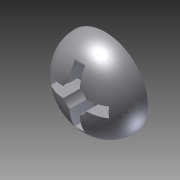
# Autodesk Inventor part: Bolt1
Saved by Autodesk Inventor 2012 SP2 (Build 160219200, 219)
## iProperties
Created: 2014-02-08
Part Number: Bolt1
Material: Default
Document SubType Name: Modeling
Designer: 1
Density: 1 g/cm^3
Author: 1
Autodesk Inventor part; units mm, degrees
ref_plane "YZ Plane" through (0, 0, 0) normal (1, 0, 0) x (0, 1, 0)
ref_plane "XZ Plane" through (0, 0, 0) normal (0, 1, 0) x (-1, 0, 0)
ref_plane "XY Plane" through (0, 0, 0) normal (0, 0, 1) x (1, 0, 0)
sketch "Sketch1" plane through (0, 0, 0) normal (0, 0, 1) x (1, 0, 0)
  circle A0 centre (-3.4351, -7.3738) radius 1.5 projected
  circle A1 centre (-3.4351, -7.3738) radius 4.4749
  point P0 (0, 0)
  constraints: 1 centre point, 1 coincident
extrude "Extrusion1" add sketch "Sketch1" along normal blind 3.175 contours A0 | A1
fillet "Fillet1" radius 3.175 1 edges at (-7.91, -7.3738, 3.175)
sketch "Sketch2" plane through (-3.4351, -7.3738, 3.175) normal (0, 0, 1) x (1, 0, 0)
  circle A0 centre (0, 0) radius 1.2999 construction
  line L0 (-6.0004, 0) -> (5.9052, 0) construction
  line L1 (0.0173, 5.7893) -> (0.0173, -4.6347) construction
  line L2 (1.1846, 0.5352) -> (3.0338, 0.5352)
  line L3 (3.0338, 0.5352) -> (3.0338, 0)
  line L4 (1.1846, -0.5352) -> (3.0338, -0.5352)
  line L5 (3.0338, -0.5352) -> (3.0338, 0)
  line L6 (-0.5352, 1.1846) -> (-0.5352, 3.0338)
  line L7 (-0.5352, 3.0338) -> (0, 3.0338)
  line L8 (0.5352, 1.1846) -> (0.5352, 3.0338)
  line L9 (0.5352, 3.0338) -> (0, 3.0338)
  line L10 (-1.1846, -0.5352) -> (-3.0338, -0.5352)
  line L11 (-3.0338, -0.5352) -> (-3.0338, 0)
  line L12 (-1.1846, 0.5352) -> (-3.0338, 0.5352)
  line L13 (-3.0338, 0.5352) -> (-3.0338, 0)
  line L14 (0.5352, -1.1846) -> (0.5352, -3.0338)
  line L15 (0.5352, -3.0338) -> (0, -3.0338)
  line L16 (-0.5352, -1.1846) -> (-0.5352, -3.0338)
  line L17 (-0.5352, -3.0338) -> (0, -3.0338)
  arc A1 (1.1846, 0.5352) -> (0.5352, 1.1846) centre (0, 0) ccw
  arc A2 (-0.5352, 1.1846) -> (-1.1846, 0.5352) centre (0, 0) ccw
  arc A3 (-1.1846, -0.5352) -> (-0.5352, -1.1846) centre (0, 0) ccw
  arc A4 (0.5352, -1.1846) -> (1.1846, -0.5352) centre (0, 0) ccw
  point P0 (3.4351, 7.3738)
  dimension "d5" = 360
  constraints: 36 end point, 10 point on circle, 4 centre point, 4 coincident, 3 perpendicular, 2 symmetric about line, 1 horizontal, 1 point on line, 37 other
extrude "Extrusion2" cut sketch "Sketch2" against normal blind 2.54
body "Solid1"
